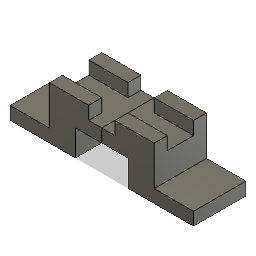
400139c2-2c31-4f76-b397-06023b9400ee (Autodesk Fusion 360 design; units mm, degrees)
Autodesk Fusion 360 part; units mm, degrees
sketch "Sketch1" plane through (0, 0, 0) normal (0, 0, 1) x (1, 0, 0)
  line L0 (-50, 0) -> (0, 0)
  line L1 (0, 0) -> (0, 20)
  line L2 (0, 20) -> (20, 20)
  line L3 (20, 20) -> (20, 30)
  line L4 (20, 30) -> (10, 30)
  line L5 (10, 30) -> (10, 40)
  line L6 (10, 40) -> (-20, 40)
  line L7 (-20, 40) -> (-20, 10)
  line L8 (-20, 10) -> (-50, 10)
  line L9 (-50, 10) -> (-50, 0)
extrude "Extrude1" add sketch "Sketch1" against normal blind 40 makes body 1
sketch "Sketch2" plane through (0, 0, 0) normal (0, 1, 0) x (1, 0, 0)
sketch "Sketch3" plane through (0, 40, 0) normal (0, 1, 0) x (-1, 0, 0)
  line L0 (20, 0) -> (-10, 0)
  line L1 (-10, 0) -> (-10, -40)
  line L2 (-10, -40) -> (20, -40)
  line L3 (20, -40) -> (20, 0)
  line L4 (20, -30) -> (-10, -30)
  line L5 (-10, -30) -> (-10, -10)
  line L6 (-10, -10) -> (20, -10)
  line L7 (20, -10) -> (20, -30)
extrude "Extrude2" cut sketch "Sketch3" against normal blind 10 contours L1 L3 L4 L5 L6 L7 bodies 1
mirror "Mirror1" about plane through (20, 20, 0) normal (1, 0, 0) of bodies 1 makes body 2
